OP Adapter Board_v1 (Autodesk Fusion 360 design; units mm, degrees)
Autodesk Fusion 360 part; units mm, degrees
sketch "Skizze1" plane through (0, 0, 0) normal (0, 0, 1) x (1, 0, 0)
  line L0 (-5.7, 4.6) -> (5.7, 4.6)
  line L1 (5.7, 4.6) -> (5.7, -4.6)
  line L2 (5.7, -4.6) -> (-5.7, -4.6)
  line L3 (-5.7, -4.6) -> (-5.7, 4.6)
  line L4 (0, 1.75) -> (0, 22.5)
  line L5 (1.75, 0) -> (22.5, 0)
  dimension "d1" = 11.4
  dimension "d2" = 9.2
  constraint horizontal L0
  constraint vertical L1
  constraint horizontal L2
  constraint vertical L3
  constraint symmetric L0 L2 L5
  measures "d1" distance of L1.end L2.end
  measures "d2" distance of L0.end L1.end
extrude "Extrusion1" add sketch "Skizze1" along normal blind 1.4
